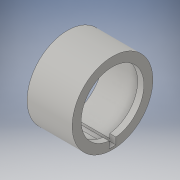
# Autodesk Inventor part: Button-NUC-Mount
Saved by Autodesk Inventor 2016 (Build 200138000, 138)
## iProperties
Created: 2015-10-16
Part Number: Button-NUC-Mount
Material: Generic
Document SubType Name: Modeling
Designer: lachesis
Density: 1 g/cm^3
Appearance: Default
Author: lachesis
Autodesk Inventor part; units mm, degrees
ref_plane "YZ Plane" through (0, 0, 0) normal (1, 0, 0) x (0, 1, 0)
ref_plane "XZ Plane" through (0, 0, 0) normal (0, 1, 0) x (-1, 0, 0)
ref_plane "XY Plane" through (0, 0, 0) normal (0, 0, 1) x (1, 0, 0)
sketch "Sketch1" plane through (0, 0, 0) normal (1, 0, 0) x (0, 1, 0)
  circle A0 centre (0, 0) radius 13
  dimension "d0" = 26
  constraints: 1 centre point, 1 coincident
  measures "d0" diameter of A0
extrude "Extrusion1" add sketch "Sketch1" along normal blind 14.5
sketch "Sketch2" plane through (0, 0, 0) normal (-1, 0, 0) x (0, 0, 1)
  circle A0 centre (0, 0) radius 13 projected
  circle A1 centre (0, 0) radius 11.5
  dimension "d3" = 23
  constraints: 1 centre point, 1 coincident
  measures "d3" diameter of A1
extrude "Extrusion2" cut sketch "Sketch2" against normal blind 12.5 contours A1
sketch "Sketch3" plane through (14.5, 0, 0) normal (1, 0, 0) x (0, 0, -1)
  circle A0 centre (0, 0) radius 13 projected
  circle A1 centre (0, 0) radius 10.1
  dimension "d6" = 20.2
  constraints: 1 centre point, 1 coincident
  measures "d6" diameter of A1
extrude "Extrusion3" cut sketch "Sketch3" against normal through all contours A1
sketch "Sketch4" plane through (14.5, 0, 0) normal (1, 0, 0) x (0, 0, -1)
  circle A0 centre (0, 0) radius 10.1 projected
  circle A1 centre (0, 0) radius 13 projected
  circle A2 centre (0, 0) radius 10.1 projected
  line L0 (-1.1, -10.0399) -> (-1.1, -12.2399)
  line L1 (-1.1, -12.2399) -> (1.1, -12.2399)
  line L2 (1.1, -12.2399) -> (1.1, -10.0399)
  dimension "d9" = 2.2
  constraints: 6 end point, 4 point on circle, 2 equal length, 2 perpendicular, 1 vertical
  measures "d9" distance of L1.end L2.end
extrude "Extrusion4" cut sketch "Sketch4" against normal through all contours A0 L2 L1 L0
body "Solid1"
